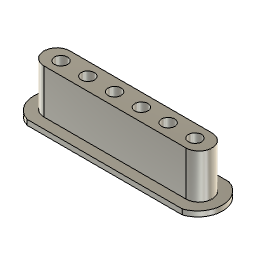
tele_rear_body v1 (Autodesk Fusion 360 design; units mm, degrees)
Autodesk Fusion 360 part; units mm, degrees
sketch "スケッチ1" plane through (0, 0, 0) normal (0, 0, 1) x (1, 0, 0)
  line L0 (0, 0) -> (72.6, 0)
  line L1 (72.6, 0) -> (72.6, -36.25)
  line L2 (72.6, -36.25) -> (0, -36.25)
  line L3 (0, -36.25) -> (0, 0)
  line L4 (36.3, 0) -> (36.3, -36.25)
  line L5 (0, -18.125) -> (72.6, -18.125)
  line L6 (72.6, -8.625) -> (72.6, -26.625)
  line L7 (58.3, -36.25) -> (14.3, -36.25)
  line L8 (0, -9.125) -> (0, -27.125)
  line L9 (0, -18.125) -> (9.5, -18.125)
  line L10 (0, -9.125) -> (6.4586, -9.125)
  line L11 (0, -27.125) -> (4.6488, -27.125)
  line L12 (6.4586, -9.125) -> (36.3, 0)
  line L13 (14.3, -36.25) -> (12.3, -36.25)
  line L14 (12.3, -36.25) -> (2.2204, -24.2289)
  line L15 (36.3, -18.125) -> (36.3, -32.425)
  line L16 (36.3, -18.125) -> (36.3, -3.825)
  line L17 (66.1414, -9.125) -> (36.3, 0)
  line L18 (60.3, -36.25) -> (70.3796, -24.2289)
  line L19 (58.3, -36.25) -> (60.3, -36.25)
  line L20 (6.4586, -27.125) -> (66.1414, -27.125)
  line L21 (6.4586, -9.125) -> (66.1414, -9.125)
  arc A0 (6.9878, -8.9632) -> (6.4586, -27.125) centre (9.5, -18.125) ccw
  arc A1 (66.1414, -27.125) -> (65.6122, -8.9632) centre (63.1, -18.125) ccw
  circle A2 centre (14.3, -32.425) radius 1.75
  circle A3 centre (36.3, -3.825) radius 1.75
  circle A4 centre (58.3, -32.425) radius 1.75
  circle A5 centre (32.3, -32.425) radius 1
  circle A6 centre (40.3, -32.425) radius 1
  point P0 (36.3, -18.125)
  point P1 (36.3, -3.825)
  point P2 (14.3, -32.425)
  point P3 (58.3, -32.425)
  point P4 (40.3, -32.425)
  point P5 (40.3, -32.425)
  point P6 (32.3, -32.425)
  dimension "d5" = 72.6
  dimension "d6" = 36.25
  dimension "d10" = 44
  dimension "d11" = 9
  dimension "d12" = 18
  dimension "d13" = 9.5
  dimension "d14" = 2
  dimension "d15" = 14.3
  dimension "d16" = 22
  dimension "d17" = 14.3
  dimension "d18" = 3.5
  dimension "d19" = 3.5
  dimension "d20" = 3.5
  dimension "d21" = 4
  dimension "d24" = 2
  dimension "d25" = 2
  constraint coincident L0.start L3.end
  constraint horizontal L0
  constraint vertical L1
  constraint horizontal L2
  constraint vertical L3
  constraint midpoint L0 L4.start
  constraint midpoint L2 L4.end
  constraint midpoint L3 L5.start
  constraint midpoint L1 L5.end
  constraint midpoint L5 P0
  constraint vertical L6
  constraint coincident L1 L6.end
  constraint parallel L2 L7
  constraint parallel L3 L8
  constraint perpendicular L8 L9
  constraint perpendicular L3 L10
  constraint perpendicular L8 L11
  constraint parallel L2 L13
  constraint coincident P0 L15.start
  constraint perpendicular L5 L15
  constraint perpendicular L0 L16
  constraint coincident P1 L16.end
  constraint symmetric L4.start L16 L12.end
  constraint symmetric L7.end L16 L7.start
  constraint symmetric L10.end L16 L17.start
  constraint symmetric L13.end L16 L18.start
  constraint symmetric L14.end L16 L18.end
  constraint perpendicular L1 L20
  constraint coincident L12 A0.start
  constraint coincident L17 A1.end
  constraint coincident L14 L11.end
  constraint coincident P2 A2.centre
  constraint coincident P3 A4.centre
  constraint coincident P6 A5.centre
  constraint coincident P5 P4
  measures "d5" distance of L0.start L0.end
  measures "d6" distance of L0.start L2.end
  measures "d10" distance of L7.start L7.end
  measures "d11" distance of L5.start L8.start
  measures "d12" distance of L8.start L8.end
  measures "d13" distance of L5.start L9.end
  measures "d14" distance of L7.end L13.end
  measures "d15" distance of P0 L15.end
  measures "d16" distance of L15.end P2
  measures "d17" distance of P0 P1
  measures "d18" diameter of A2
  measures "d19" diameter of A3
  measures "d20" diameter of A4
  measures "d21" distance of L15.end P5
  measures "d24" diameter of A5
  measures "d25" diameter of A6
extrude "押し出し2" add sketch "スケッチ1" along normal blind 19 contours L4 L5 L9 L16 L21 A0 | L4 L5 L9 L15 L20 A0 | L4 L5 L16 L21 A1 | L4 L5 L15 L20 A1
sketch "スケッチ3" plane through (0, 0, 0) normal (0, 0, -1) x (1, 0, 0)
  arc A0 (6.4586, 27.125) -> (6.4586, 9.125) centre (9.5, 18.125) ccw
  line L0 (6.4586, 9.125) -> (66.1414, 9.125)
  arc A1 (66.1414, 9.125) -> (66.1414, 27.125) centre (63.1, 18.125) ccw
  line L1 (66.1414, 27.125) -> (6.4586, 27.125)
  line L2 (72.6, 18.125) -> (0, 18.125)
  line L3 (72.6, 18.125) -> (36.3, 18.125)
  line L4 (36.3, 18.125) -> (31.15, 18.125)
  line L5 (31.15, 18.125) -> (20.85, 18.125)
  line L6 (20.85, 18.125) -> (10.55, 18.125)
  line L7 (36.3, 18.125) -> (36.3, 27.125)
  point P0 (36.3, 18.125)
  point P1 (31.15, 18.125)
  point P2 (20.85, 18.125)
  point P3 (10.55, 18.125)
  point P4 (41.45, 18.125)
  point P5 (51.75, 18.125)
  point P6 (62.05, 18.125)
  dimension "d32" = 5.15
  dimension "d33" = 10.3
  dimension "d34" = 10.3
  constraint midpoint A1 L2.start
  constraint midpoint A0 L2.end
  constraint midpoint L2 P0
  constraint coincident P0 L3.end
  constraint coincident L2 P1
  constraint parallel L2 L5
  constraint coincident L2 P3
  constraint coincident P1 L4.end
  constraint coincident P2 L5.end
  constraint coincident P3 L6.end
  constraint midpoint L1 L7.end
  constraint symmetric P1 L7 P4
  constraint symmetric P2 L7 P5
  constraint symmetric P3 L7 P6
  measures "d32" distance of P0 P1
  measures "d33" distance of P1 P2
  measures "d34" distance of P2 P3
hole "穴1" at (62.05, -18.125, 0) at (51.75, -18.125, 0) at (41.45, -18.125, 0) at (31.15, -18.125, 0) at (20.85, -18.125, 0) at (10.55, -18.125, 0) direction (0, 0, 1) diameter 5 depth 23 tip angle 180
sketch "スケッチ4" plane through (0, 0, 19) normal (0, 0, 1) x (-1, 0, 0)
  circle A0 centre (-20.85, 18.125) radius 2.5
  circle A1 centre (-41.45, 18.125) radius 2.5
  circle A2 centre (-62.05, 18.125) radius 2.5
  circle A3 centre (-51.75, 18.125) radius 2.5
  circle A4 centre (-31.15, 18.125) radius 2.5
  circle A5 centre (-10.55, 18.125) radius 2.5
  arc A6 (-6.4586, 9.125) -> (-6.4586, 27.125) centre (-9.5, 18.125) ccw
  line L0 (-6.4586, 27.125) -> (-66.1414, 27.125)
  arc A7 (-66.1414, 27.125) -> (-66.1414, 9.125) centre (-63.1, 18.125) ccw
  line L1 (-66.1414, 9.125) -> (-6.4586, 9.125)
  line L2 (0, 18.125) -> (-4, 18.125)
  line L3 (-36.3, 13.125) -> (-5.4223, 13.125)
  line L4 (-4, 18.125) -> (-13.5, 18.125)
  line L5 (-36.3, 23.125) -> (-5.4223, 23.125)
  line L6 (-36.3, 23.125) -> (-36.3, 27.125)
  arc A8 (-5.4223, 13.125) -> (-5.4223, 23.125) centre (-13.5, 18.125) ccw
  line L7 (-36.3, 13.125) -> (-67.1777, 13.125)
  arc A9 (-67.1777, 23.125) -> (-67.1777, 13.125) centre (-59.1, 18.125) ccw
  line L8 (-36.3, 23.125) -> (-67.1777, 23.125)
  line L9 (-36.3, 23.125) -> (-36.3, 13.125)
  line L10 (-31.15, 18.125) -> (-41.45, 18.125)
  point P0 (-68.6, 18.125)
  dimension "d39" = 9.5
  dimension "d40" = 4
  dimension "d45" = 4
  dimension "d46" = 5
  dimension "d47" = 9.5
  dimension "d48" = 10.3
  constraint midpoint A6 L2.start
  constraint horizontal L2
  constraint midpoint L0 L6.end
  constraint horizontal L4
  constraint symmetric L2.end L6 P0
  constraint symmetric L3.start L6 L7.start
  constraint symmetric L5.start L6 L8.start
  constraint symmetric L6 L3.end L7.end
  constraint symmetric L6 L5.end A9.start
  constraint symmetric L6 A8 A9
  constraint perpendicular L7 L9
  constraint coincident A4.centre L10.start
  constraint coincident A1.centre L10.end
  measures "d39" distance of L2.end L4.end
  measures "d40" distance of L6.end L5.start
  measures "d45" distance of L2.start L2.end
  measures "d46" diameter of A4
  measures "d47" radius of A8
  measures "d48" distance of A4.centre A1.centre
extrude "押し出し3" cut sketch "スケッチ4" against normal blind 17 contours A6 L0 A7 L1 L2 L3 L6 A8 L7 A9 L8 | A6 L0 L2 L5 L6 A8
fillet "フィレット2" radius 5 4 edges at (5.4223, -23.125, 10.5) (5.4223, -13.125, 10.5) (67.1777, -13.125, 10.5) (67.1777, -23.125, 10.5)
